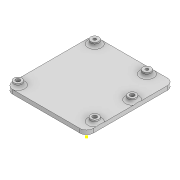
# Autodesk Inventor part: Electronics_mount
Saved by Autodesk Inventor 2022 (Build 260153000, 153)
## iProperties
Created: 2022-09-21
Part Number: Electronics_mount
Material: Generic
Document SubType Name: Modeling
Designer: dell
Density: 1 g/cm^3
Appearance: Default
Author: dell
Autodesk Inventor part; units mm, degrees
ref_plane "YZ Plane" through (0, 0, 0) normal (1, 0, 0) x (0, 1, 0)
ref_plane "XZ Plane" through (0, 0, 0) normal (0, 1, 0) x (-1, 0, 0)
ref_plane "XY Plane" through (0, 0, 0) normal (0, 0, 1) x (1, 0, 0)
sketch "Sketch1" plane through (0, 0, 0) normal (0, 1, 0) x (-1, 0, 0)
  line L0 (0, 0) -> (60, 0)
  line L1 (60, 0) -> (60, -65)
  line L2 (60, -65) -> (0, -65)
  line L3 (0, -65) -> (0, 0)
  circle A0 centre (4, -10) radius 1.55
  circle A1 centre (4, -37.94) radius 1.55
  circle A2 centre (56.07, -4.92) radius 1.55
  circle A3 centre (56.07, -4.92) radius 3
  circle A4 centre (4, -10) radius 3
  circle A5 centre (4, -37.94) radius 3
  circle A6 centre (54, -60) radius 1.05
  circle A7 centre (54, -60) radius 3
  circle A8 centre (15.138, -60) radius 1.05
  circle A9 centre (15.138, -60) radius 3
  dimension "d0" = 60
  dimension "d1" = 65
  dimension "d4" = 3.1
  dimension "d5" = 10
  dimension "d6" = 3.1
  dimension "d8" = 4
  dimension "d9" = 3.1
  dimension "d10" = 52.07
  dimension "d11" = 5.08
  dimension "d12" = 27.94
  dimension "d13" = 6
  dimension "d14" = 6
  dimension "d15" = 6
  dimension "d18" = 2.1
  dimension "d19" = 60
  dimension "d20" = 54
  dimension "d21" = 6
  dimension "d22" = 2.1
  dimension "d23" = 6
  dimension "d24" = 38.862
  constraints: 10 centre point, 8 end point, 5 coincident, 2 parallel, 1 horizontal, 1 horizontal alignment, 1 perpendicular, 1 vertical alignment
  measures "d0" distance between parallel lines of L1 L3
  measures "d1" distance between parallel lines of L2 L0
  measures "d4" diameter of A0
  measures "d5" distance from line of L0 A0.centre
  measures "d6" diameter of A1
  measures "d8" distance from line of L3 A0.centre
  measures "d9" diameter of A2
  measures "d10" horizontal distance of A0.centre A2.centre
  measures "d11" vertical distance of A0.centre A2.centre
  measures "d12" distance of A1.centre A0.centre
  measures "d13" diameter of A3
  measures "d14" diameter of A4
  measures "d15" diameter of A5
  measures "d18" diameter of A6
  measures "d19" distance from line of L0 A6.centre
  measures "d20" distance from line of L3 A6.centre
  measures "d21" diameter of A7
  measures "d22" diameter of A8
  measures "d23" diameter of A9
  measures "d24" distance of A6.centre A8.centre
extrude "Extrusion1" add sketch "Sketch1" along normal blind 3 contours L0 L1 L2 L3 | A3 | A4 | A5 | A7 | A9
extrude "Extrusion2" add sketch "Sketch1" along normal blind 6 contours A3 | A4 | A5 | A7 | A9
fillet "Fillet1" radius 2 5 edges at (-53.07, 3, -4.92) (-1, 3, -10) (-1, 3, -37.94) (-12.138, 3, -60) (-51, 3, -60)
sketch "Sketch2" plane through (0, 0, 0) normal (0, -1, 0) x (1, 0, 0)
  line L0 (-35.4, -18) -> (-38.4, -18)
  line L1 (-38.4, -18) -> (-38.4, -47)
  line L2 (-38.4, -47) -> (-35.4, -47)
  line L3 (-35.4, -47) -> (-35.4, -18)
  line L4 (0, 0) -> (0, -65) projected
  line L5 (-60, 0) -> (0, 0) projected
  line L6 (0, -65) -> (-60, -65) projected
  line L7 (-41.4, -18) -> (-44.4, -18)
  line L8 (-44.4, -18) -> (-44.4, -47)
  line L9 (-44.4, -47) -> (-41.4, -47)
  line L10 (-41.4, -47) -> (-41.4, -18)
  line L11 (-60, -65) -> (-60, 0) projected
  dimension "d26" = 3
  dimension "d28" = 18
  dimension "d29" = 18
  dimension "d30" = 3
  dimension "d31" = 3
  dimension "d54" = 15.6
  constraints: 16 end point, 4 parallel, 2 collinear, 2 horizontal, 2 perpendicular
  measures "d26" distance between parallel lines of L3 L1
  measures "d28" distance between parallel lines of L5 L0
  measures "d29" distance between parallel lines of L6 L2
  measures "d30" distance between parallel lines of L1 L10
  measures "d31" distance between parallel lines of L8 L10
  measures "d54" distance between parallel lines of L11 L8
extrude "Extrusion3" add sketch "Sketch2" along normal blind 8 contours L3 L2 L1 L0 | L10 L9 L8 L7
sketch "Sketch3" plane through (-35.4, 0, -18) normal (1, 0, 0) x (0, 0, -1)
  circle A0 centre (4.5, -4.3) radius 1.55
  circle A1 centre (24.5, -4.3) radius 1.55
  line L0 (0, 0) -> (0, -8) projected
  line L1 (29, 0) -> (29, -8) projected
  line L2 (-18, 0) -> (47, 0) projected
  dimension "d34" = 3.1
  dimension "d35" = 3.1
  dimension "d36" = 4.5
  dimension "d37" = 4.5
  dimension "d38" = 4.3
  dimension "d39" = 4.3
  constraints: 2 centre point
  measures "d34" diameter of A0
  measures "d35" diameter of A1
  measures "d36" distance from line of L0 A0.centre
  measures "d37" distance from line of L1 A1.centre
  measures "d38" distance from line of L2 A0.centre
  measures "d39" distance from line of L2 A1.centre
extrude "Extrusion4" cut sketch "Sketch3" against normal blind 10
thicken "Thicken1" operation add thickness 0.15 both sides no extend neighbours yes toward (1, 0, 0) faces at (-38.4, -0.9502, -29.3499)
thicken "Thicken2" operation add thickness 0.15 both sides no extend neighbours yes toward (-1, 0, 0) faces at (-41.4, -0.9502, -35.6501)
chamfer "Chamfer1" distance 8 angle 45 4 edges at (-36.825, 0, -18) (-42.975, 0, -18) (-36.825, 0, -47) (-42.975, 0, -47)
fillet "Fillet2" radius 5 4 edges at (0, 1.5, -65) (-60, 1.5, -65) (-60, 1.5, 0) (0, 1.5, 0)
fillet "Fillet3" radius 1 2 edges at (-35.4, 0, -32.5) (-44.4, 0, -32.5)
sketch "Sketch4" plane through (0, 0, 0) normal (0, -1, 0) x (1, 0, 0)
  point P0 (0, 0)
body "Solid1"
